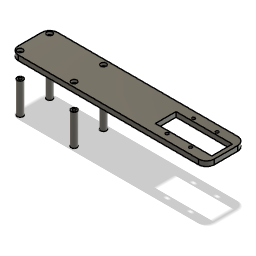
_Center Arm Top.5e4394fa-e90c-437b-a858-13c8ca8d634e (Autodesk Fusion 360 design; units mm, degrees)
Autodesk Fusion 360 part; units mm, degrees
note: some values were not read from the file. Chosen so that the rebuilt part matches the saved one: which bodies a step acts on; which face or edge a step refers to.
sketch "Sketch1" plane through (0, 0, 0) normal (0, 1, 0) x (1, 0, 0)
  circle A0 centre (-70, -15) radius 1.5
  line L0 (-75, 20) -> (-75, -20)
  line L1 (75, 20) -> (-75, -20) construction
  circle A1 centre (-15, -15) radius 1.5
  circle A2 centre (52.4046, 13.5) radius 1.5
  line L2 (75, 20) -> (-75, 20)
  line L3 (-75, 20) -> (75, -20) construction
  circle A3 centre (52.4046, -13.5) radius 1.5
  line L4 (-75, -20) -> (75, -20)
  line L5 (28.4046, 13.5) -> (52.4046, -13.5) construction
  line L6 (28.4046, -13.5) -> (52.4046, -13.5) construction
  line L7 (75, -20) -> (75, 20)
  line L8 (26.4996, -10.5) -> (54.3096, -10.5)
  circle A4 centre (28.4046, 13.5) radius 1.5
  line L9 (54.3096, 10.5) -> (26.4996, 10.5)
  circle A5 centre (-70, 15) radius 1.25
  line L10 (52.4046, 13.5) -> (28.4046, -13.5) construction
  circle A6 centre (28.4046, -13.5) radius 1.5
  circle A7 centre (-15, 15) radius 1.5
  line L11 (52.4046, 13.5) -> (28.4046, 13.5) construction
  line L12 (52.4046, -13.5) -> (52.4046, 13.5) construction
  line L13 (28.4046, 13.5) -> (28.4046, -13.5) construction
  line L14 (-67, 18) -> (-73, 12) construction
  line L15 (-73, 18) -> (-67, 12) construction
  circle A8 centre (-70, 15) radius 3
  circle A9 centre (-15, 15) radius 3
  circle A10 centre (-70, -15) radius 3
  circle A11 centre (-15, -15) radius 3
  line L16 (26.4996, 10.5) -> (13.5, 10.5)
  line L17 (13.5, 10.5) -> (13.5, -10.5)
  line L18 (13.5, -10.5) -> (26.4996, -10.5)
  line L19 (54.3096, 10.5) -> (71, 10.5)
  line L20 (71, 10.5) -> (71, -10.5)
  line L21 (71, -10.5) -> (54.3096, -10.5)
  point P0 (40.4046, 0)
  point P1 (-70, 15)
  dimension "d5" = -24
  dimension "d6" = 27
  dimension "d11" = 150
  dimension "d12" = 40
  dimension "d13" = 27.81
  dimension "d14" = 24
  dimension "d15" = 27
  dimension "d16" = 3
  dimension "d18" = 2.5
  dimension "d21" = 55
  dimension "d22" = -30
  constraint horizontal L2
  constraint perpendicular L0 L2
  constraint parallel L2 L4
  constraint parallel L0 L7
  constraint coincident origin L1
  constraint coincident origin L3
  constraint horizontal L11
  constraint perpendicular L11 L13
  constraint parallel L6 L11
  constraint parallel L12 L13
  constraint coincident P0 L10
  constraint coincident P0 L5
  constraint coincident L5.start A4.centre
  constraint coincident L14 P1
  constraint coincident L15 P1
  constraint concentric A5 A8
  constraint perpendicular L9 L17
  constraint parallel L9 L19
  constraint perpendicular L9 L20
  measures "d11" distance of L0.end L3.end
  measures "d12" distance of L0.end L0.start
  measures "d13" distance of L9.start L9.end
  measures "d14" distance of L6.start A3.centre
  measures "d15" distance of L6.start L5.start
  measures "d16" diameter of A4
  measures "d18" diameter of A5
extrude "Extrude1" add sketch "Sketch1" along normal blind 5 contours L0 L2 L4 L7 | A8 | A9 | A10 | A11 makes body 1
extrude "Extrude2" add sketch "Sketch1" against normal blind 32 contours A8 | A9 | A10 | A11 bodies 1
fillet "Fillet2" radius 8 4 edges at (-75, 2.5, 20) (-75, 2.5, -20) (75, 2.5, 20) (75, 2.5, -20) on bodies 1
split "Split1" by plane through (0, 0, 0) normal (1, 0, 0) bodies 1 makes body 2 at (4.5, 5, -3.5)
move_body "Move1" bodies 2 to x (1, 0, 0) y (0, 1, 0) z (0, 0, 1) at (50, 0, 0)
extrude "Extrude3" add 1 faces at (0, 3.3333, -6.6667) along direction (1, 0, 0) blind 50 on bodies 1 bodies 1 2
sketch "Sketch2" plane through (0, 5, 0) normal (0, 1, 0) x (-1, 0, 0)
  line L0 (-63.5, -10.5) -> (-121, -10.5)
  line L1 (-121, -10.5) -> (-121, 10.5)
  line L2 (-121, 10.5) -> (-104.3096, 10.5)
  line L3 (-104.3096, 10.5) -> (-76.4996, 10.5)
  line L4 (-76.4996, 10.5) -> (-63.5, 10.5)
  line L5 (-63.5, 10.5) -> (-63.5, -10.5)
  circle A0 centre (-102.4046, 13.5) radius 1.5
  circle A1 centre (-102.4046, -13.5) radius 1.5
  circle A2 centre (-78.4046, -13.5) radius 1.5
  circle A3 centre (-78.4046, 13.5) radius 1.5
  circle A4 centre (15, -15) radius 1.5
  circle A5 centre (70, 15) radius 1.5
  circle A6 centre (70, -15) radius 1.25
  circle A7 centre (15, 15) radius 1.5
  line L6 (-50, -20) -> (67, -20)
  arc A8 (67, -20) -> (75, -12) centre (67, -12) ccw
  line L7 (75, -12) -> (75, 12)
  arc A9 (75, 12) -> (67, 20) centre (67, 12) ccw
  line L8 (67, 20) -> (-50, 20)
  line L9 (-50, 20) -> (-117, 20)
  arc A10 (-117, 20) -> (-125, 12) centre (-117, 12) ccw
  line L10 (-125, 12) -> (-125, -12)
  arc A11 (-125, -12) -> (-117, -20) centre (-117, -12) ccw
  line L11 (-117, -20) -> (-50, -20)
  circle A12 centre (70, -15) radius 2.8
  circle A13 centre (15, -15) radius 2.8
  circle A14 centre (70, 15) radius 2.8
  circle A15 centre (15, 15) radius 2.8
  dimension "d33" = 5.6
  dimension "d36" = -55
  dimension "d37" = 30
  constraint concentric A6 A12
  measures "d33" diameter of A12
extrude "Extrude4" cut sketch "Sketch2" against normal blind 3 contours A12 | A13 | A14 | A15 bodies 1
split "Split2" by plane through (0, 0, 0) normal (0, 1, 0) bodies 1 makes body 3 at (-12.0037, -21.3333, 15.1495) makes body 4 at (-70.5209, -21.3333, 12.0456) makes body 5 at (-12.0037, -21.3333, -14.8505) makes body 6 at (12.5585, 5, -4.7249)
move_body "Move2" bodies 4 1 3 5 to x (1, 0, 0) y (0, 1, 0) z (0, 0, 1) at (0, -20, 0)
